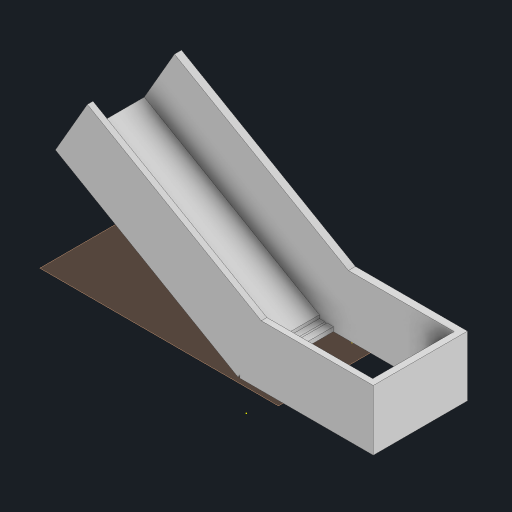
# Autodesk Inventor part: channel
Saved by Autodesk Inventor 2024 (Build 280153000, 153)
## iProperties
Created: 2023-11-07
Part Number: channel
Material: Generic
Document SubType Name: Modeling
Designer: 91840
Density: 1 g/cm^3
Appearance: Default
Author: 91840
Autodesk Inventor part; units mm, degrees
ref_plane "YZ Plane" through (0, 0, 0) normal (1, 0, 0) x (0, 1, 0)
ref_plane "XY Plane" through (0, 0, 0) normal (0, 0, 1) x (1, 0, 0)
sketch "Sketch1" plane through (0, 0, 0) normal (0, 0, 1) x (1, 0, 0)
  line L0 (-135.8451, 94.4022) -> (-5.8451, 19.3467)
  line L1 (-134.5951, 96.5673) -> (-4.5951, 21.5118)
  line L2 (-4.5951, 21.5118) -> (-5.8451, 19.3467)
  line L3 (-134.5951, 96.5673) -> (-135.8451, 94.4022)
  line L4 (-164.6473, 0) -> (36.9683, 0) projected
  point P0 (0, 0)
  dimension "d0" = 2.5
  dimension "d3" = 130
  dimension "d4" = 30
  constraints: 8 end point, 2 perpendicular, 1 other
  measures "d0" distance between parallel lines of L1 L0
  measures "d3" horizontal distance of L1.start L1.end
  measures "d4" angle to the sketch x axis of L0
extrude "Extrusion1" add sketch "Sketch1" along normal blind 67
sketch "Sketch2" plane through (-134.5951, 96.5673, 67) normal (0.5, 0.866, 0) x (0.866, -0.5, 0)
  point P0 (164.8464, 67)
sketch "Sketch4" plane through (0, 0, 67) normal (0, 0, 1) x (1, 0, 0)
  point P0 (0, 0)
sketch "Sketch5" plane through (-134.5951, 96.5673, 67) normal (0.5, 0.866, 0) x (0.866, -0.5, 0)
  line L0 (0, 67) -> (0, 0) projected
  line L1 (0, 0) -> (152, 0)
  line L2 (152, 0) -> (152, 4)
  line L3 (152, 4) -> (0, 4)
  line L4 (0, 4) -> (0, 0)
  point P0 (164.8464, 67)
  point P1 (0, 4)
  constraints: 8 end point, 2 parallel, 1 horizontal, 1 perpendicular
sketch "Sketch6" plane through (-134.5951, 96.5673, 67) normal (0.5, 0.866, 0) x (0.866, -0.5, 0)
  line L0 (0, 67) -> (150.1111, 67) projected
  line L1 (0, 67) -> (150.1111, 67)
  line L2 (150.1111, 67) -> (150.1111, 62)
  line L3 (150.1111, 62) -> (0, 62)
  line L4 (0, 62) -> (0, 67)
  point P0 (164.8464, 67)
  constraints: 8 end point, 2 parallel, 1 horizontal, 1 perpendicular
extrude "Extrusion2" add sketch "Sketch5" along normal blind 43
extrude "Extrusion3" add sketch "Sketch6" along normal blind 43
ref_plane "Work Plane1" through (0, 19.347, 0) normal (0, 1, 0) x (-1, 0, 0)
sketch "Sketch8" plane through (0, 19.347, 0) normal (0, 1, 0) x (-1, 0, 0)
  line L0 (5.8451, 67) -> (4.5951, 67) projected
  line L1 (4.5951, 67) -> (-90.4049, 67)
  line L2 (-90.4049, 67) -> (-90.4049, 0)
  line L3 (-90.4049, 0) -> (4.5951, 0)
  line L4 (4.5951, 0) -> (4.5951, 67)
  point P0 (0, 0)
  dimension "d10" = 95
  constraints: 8 end point, 2 parallel, 1 horizontal, 1 perpendicular
  measures "d10" distance of L3.end L2.end
extrude "Extrusion4" add sketch "Sketch8" along normal blind 43
sketch "Sketch9" plane through (0, 62.347, 0) normal (0, 1, 0) x (1, 0, 0)
  line L0 (-113.0951, -5) -> (10.6762, -5) projected
  line L1 (0, -5) -> (86, -5)
  line L2 (86, -5) -> (86, -63)
  line L3 (86, -63) -> (0, -63)
  line L4 (0, -63) -> (0, -5)
  point P0 (0, 0)
  constraints: 8 end point, 2 parallel, 1 horizontal, 1 perpendicular, 1 point on line
extrude "Extrusion5" cut sketch "Sketch9" against normal through all
sketch "Sketch12" plane through (0, 62.347, 63) normal (1, 0, 0) x (0, 0, -1)
  line L0 (-4, 0) -> (0, 0) projected
  line L1 (58, 0) -> (58, -43) projected
  line L2 (0, 0) -> (58, 0)
  line L3 (58, 0) -> (58, -40)
  line L4 (58, -40) -> (0, -40)
  line L5 (0, -40) -> (0, 0)
  point P0 (63, -62.347)
  constraints: 8 end point, 2 parallel, 1 horizontal, 1 perpendicular, 1 point on line
extrude "Extrusion6" cut sketch "Sketch12" against normal blind 10
body "Solid1"
